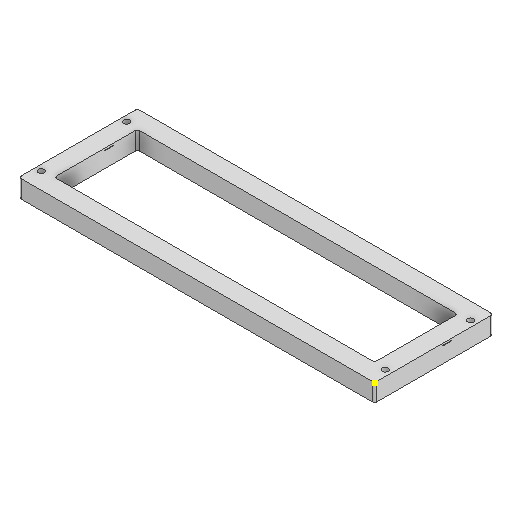
# Autodesk Inventor part: podstawka_prowadzaca
Saved by Autodesk Inventor 2025.1 (Build 291241000, 241)
## iProperties
Created: 2025-03-27
Part Number: podstawka_prowadzaca
Material: Ogólny
Document SubType Name: Modeling
Designer: Maciej
Density: 1 g/cm^3
Appearance: Domyślna
Author: Maciej
Autodesk Inventor part; units mm, degrees
ref_plane "YZ Plane" through (0, 0, 0) normal (1, 0, 0) x (0, 1, 0)
ref_plane "XZ Plane" through (0, 0, 0) normal (0, 1, 0) x (-1, 0, 0)
ref_plane "XY Plane" through (0, 0, 0) normal (0, 0, 1) x (1, 0, 0)
sketch "Szkic1" plane through (0, 0, 0) normal (0, 1, 0) x (-1, 0, 0)
  line L0 (0, 0) -> (300, 0)
  line L1 (300, 0) -> (300, -100)
  line L2 (300, -100) -> (0, -100)
  line L3 (0, -100) -> (0, 0)
  dimension "d0" = 100
  dimension "d1" = 300
  constraints: 8 end point, 2 parallel, 1 horizontal, 1 perpendicular
  measures "d0" distance of L0.end L1.end
  measures "d1" distance of L1.end L2.end
sketch "Szkic2" plane through (0, 0, 0) normal (0, 1, 0) x (-1, 0, 0)
  line L0 (15, -15) -> (285, -15)
  line L1 (285, -15) -> (285, -85)
  line L2 (285, -85) -> (15, -85)
  line L3 (15, -85) -> (15, -15)
  point P0 (0, 0)
  dimension "d2" = 270
  dimension "d3" = 70
  dimension "d4" = 15
  dimension "d5" = 15
  constraints: 8 end point, 2 parallel, 1 horizontal, 1 perpendicular
  measures "d2" distance of L1.end L2.end
  measures "d3" distance of L0.end L1.end
  measures "d4" horizontal distance of point (0, 0) L0.start
  measures "d5" horizontal distance of point (0, 0) L0.start
extrude "Wyciągnięcie proste1" add sketch "Szkic1" along normal blind 15
extrude "Wyciągnięcie proste2" cut sketch "Szkic2" along normal blind 15
fillet "Zaokrąglenie1" radius 2 8 edges at (-285, 7.5, -85) (-15, 7.5, -85) (-15, 7.5, -15) (-285, 7.5, -15) (-300, 7.5, 0) (-300, 7.5, -100) (0, 7.5, -100) (0, 7.5, 0)
sketch "Szkic3" plane through (0, 15, 0) normal (0, 1, 0) x (1, 0, 0)
  line L0 (0, 2) -> (0, 98) projected
  line L1 (-2, 100) -> (-298, 100) projected
  line L2 (-298, 0) -> (-2, 0) projected
  line L3 (-300, 98) -> (-300, 2) projected
  point P0 (0, 0)
  point P1 (-5, 86)
  point P2 (-5, 14)
  point P3 (-295, 86)
  point P4 (-295, 14)
  dimension "d11" = 5
  dimension "d12" = 14
  dimension "d13" = 14
  dimension "d14" = 14
  dimension "d15" = 5
  dimension "d16" = 5
  dimension "d17" = 5
  dimension "d18" = 14
  measures "d11" distance from line of L0 point (-5, 86)
  measures "d12" distance from line of L1 point (-5, 86)
  measures "d13" distance from line of L2 point (-5, 14)
  measures "d14" distance from line of L2 point (-295, 14)
  measures "d15" distance from line of L0 point (-5, 14)
  measures "d16" distance from line of L3 point (-295, 14)
  measures "d17" distance from line of L3 point (-295, 86)
  measures "d18" distance from line of L1 point (-295, 86)
hole "Otwór1" at (-5, 15, -86) at (-5, 15, -14) at (-295, 15, -86) at (-295, 15, -14) direction (0, -1, 0) diameter 5 depth 15 clearance for "Śruba ze łbem płaskim obrobiona" size "M4" standard "ANSI Profil metryczny M"
sketch "Szkic4" plane through (0, 15, 0) normal (0, 1, 0) x (1, 0, 0)
  point P0 (0, 0)
sketch "Szkic5" plane through (0, 0, -2) normal (1, 0, 0) x (0, 0, -1)
  line L0 (55.525, 13.5) -> (62.525, 13.5)
  line L1 (62.525, 13.5) -> (62.525, 13)
  line L2 (62.525, 13) -> (55.525, 13)
  line L3 (55.525, 13) -> (55.525, 13.5)
  line L4 (0, 15) -> (96, 15) projected
  line L5 (98, 0) -> (98, 15) projected
  point P0 (-2, 0)
  point P1 (62.525, 13.25)
  dimension "d26" = 7
  dimension "d27" = 0.5
  dimension "d28" = 1.5
  dimension "d29" = 35.475
  constraints: 8 end point, 2 parallel, 1 horizontal, 1 midpoint, 1 perpendicular
  measures "d26" distance of L1.end L2.end
  measures "d27" distance of L0.end L1.end
  measures "d28" distance between parallel lines of L4 L0
  measures "d29" distance from line of L5 point (62.525, 13.25)
extrude "Wyciągnięcie proste3" cut sketch "Szkic5" against normal through all
equation "\"d13\" = d12"
equation "\"d14\" = d12"
equation "\"d15\" = d11"
equation "\"d16\" = d11"
equation "\"d17\" = d11"
equation "\"d18\" = d12"
